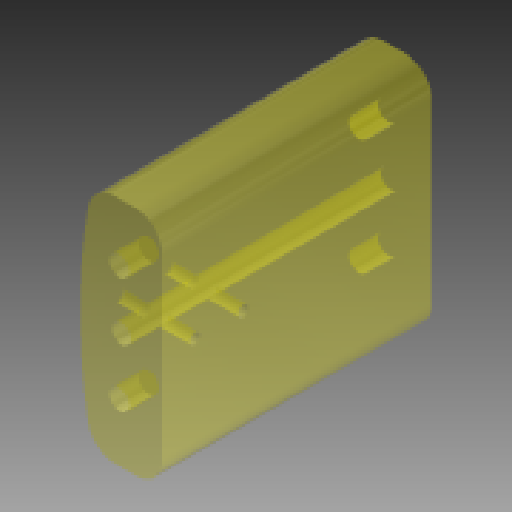
# Autodesk Inventor part: крепление ручки
Saved by Autodesk Inventor 2023 (Build 270158000, 158)
## iProperties
Created: 2025-04-14
Part Number: крепление ручки
Material: Типовые
Document SubType Name: Modeling
Designer: Ivan
Density: 1 g/cm^3
Appearance: Прозрачный — желтый
Author: Ivan
Autodesk Inventor part; units mm, degrees
ref_plane "YZ Plane" through (0, 0, 0) normal (1, 0, 0) x (0, 1, 0)
ref_plane "XZ Plane" through (0, 0, 0) normal (0, 1, 0) x (-1, 0, 0)
ref_plane "XY Plane" through (0, 0, 0) normal (0, 0, 1) x (1, 0, 0)
ref_plane "РабПлоскость1" through (0, 0, 0) normal (0, 0, 1) x (1, 0, 0)
sketch "Эскиз1" plane through (0, 0, 0) normal (0, 0, 1) x (1, 0, 0)
  arc A0 (-36.9892, 97.1998) -> (-36.9892, -97.1998) centre (0, 0) ccw projected
  line L0 (-145.6, 0) -> (145.6, 0) construction
  line L1 (-101.7534, 21.5) -> (-88.7534, 21.5)
  line L2 (-88.7534, 21.5) -> (-88.7534, -21.5)
  line L3 (-88.7534, -21.5) -> (-101.7534, -21.5)
  line L4 (-101.7534, -21.5) -> (-101.7534, 21.5) construction
  line L5 (-104, 0) -> (-88.7534, 0) construction
  circle A1 centre (-96.3767, 0) radius 1.75
  point P0 (0, 0)
  point P1 (-101.7534, 0)
  point P2 (-101.7534, 21.5)
  dimension "d0" = 43
  dimension "d1" = 13
  dimension "d2" = 3.5
  constraints: 12 end point, 3 midpoint, 2 horizontal, 2 parallel, 2 point on circle, 2 point on line, 1 centre point, 1 perpendicular, 2 other
  measures "d0" distance of L3.end L1.start
  measures "d1" distance of L2.end L3.end
  measures "d2" diameter of A1
ref_plane "РабПлоскость2" through (-75.9237, -75.9237, 50) normal (0, 0, 1) x (0.7071068, -0.7071068, 0)
extrude "Выдавливание1" add sketch "Эскиз1" along normal up to surface (50 mm away)
fillet "Сопряжение1" radius 5 4 edges at (-101.7534, 21.5, 25) (-88.7534, 21.5, 25) (-88.7534, -21.5, 25) (-101.7534, -21.5, 25)
sketch "Эскиз2" plane through (-88.7534, -16.5, 0) normal (1, 0, 0) x (0, 0, -1)
  line L0 (-50, 18.25) -> (-50, 14.75) projected
  line L1 (0, 14.75) -> (0, 18.25) projected
  circle A0 centre (-44, 16.5) radius 1
  line L2 (-50, 14.75) -> (0, 14.75) projected
  circle A1 centre (-35, 16.5) radius 1
  line L3 (-50, 16.5) -> (0, 16.5) construction
  line L4 (-50, 33) -> (-50, 0) projected
  point P0 (0, 16.5)
  dimension "d6" = 2
  dimension "d9" = 6
  dimension "d10" = 15
  constraints: 3 midpoint, 2 centre point, 2 end point, 2 point on line, 1 equal radius
  measures "d6" diameter of A0
  measures "d9" distance from line of A0.centre L4
  measures "d10" distance from line of A1.centre L4
extrude "Выдавливание2" cut sketch "Эскиз2" against normal through all
chamfer "Фаска1" distance 1.3 angle 45 2 edges at (-104, 0.0084, 45) (-104, 0.0084, 36)
sketch "Эскиз3" plane through (-97.6153, -21.5, 50) normal (0, 0, 1) x (1, 0, 0)
  line L0 (0.8568, 43) -> (0.8568, 0) construction
  circle A0 centre (0.8568, 21.5) radius 1.8 projected
  line L1 (0, 43) -> (3.8619, 43) construction
  line L2 (3.8619, 0) -> (0, 0) construction
  circle A1 centre (0.8568, 32.25) radius 1.9
  circle A2 centre (0.8568, 10.75) radius 1.9
  point P0 (97.6153, 21.5)
  point P1 (0.8568, 21.5)
  dimension "d16" = 21.5
  dimension "d17" = 10.75
  dimension "d18" = 10.75
  dimension "d19" = 3.8
  constraints: 4 point on line, 3 coincident, 2 centre point, 2 end point, 2 midpoint, 1 equal radius, 1 vertical
  measures "d16" distance from line of point (0.857, 21.5) L1
  measures "d17" distance from line of point (0.857, 32.25) L1
  measures "d18" distance from line of point (0.857, 10.75) L2
  measures "d19" diameter of A1
extrude "Выдавливание3" cut sketch "Эскиз3" against normal blind 5.5 contours A1 | A2
ref_plane "РабПлоскость3" through (-97.6153, -21.5, 25) normal (0, 0, 1) x (1, 0, 0)
mirror "Зеркальное отражение1" about plane through (-97.6153, -21.5, 25) normal (0, 0, 1) of "Выдавливание3"
equation "\"d17\" = 0.5 * d16"
equation "\"d18\" = d17"
